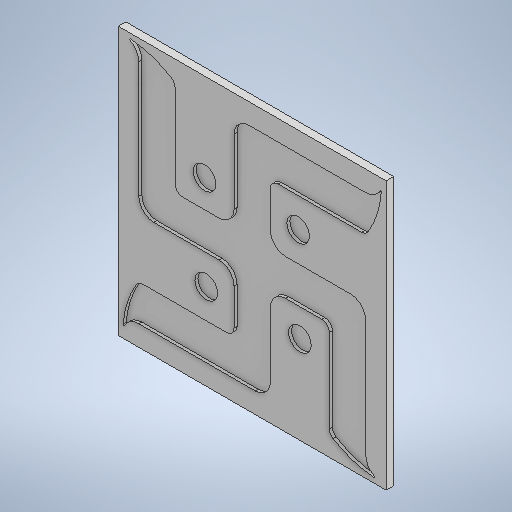
# Autodesk Inventor part: swastik@2
Saved by Autodesk Inventor 2025.2 (Build 292293000, 293)
## iProperties
Created: 2025-04-25
Part Number: swastik@2
Material: Generic
Document SubType Name: Modeling
Designer: spars
Density: 1 g/cm^3
Appearance: Default
Author: spars
Autodesk Inventor part; units mm, degrees
ref_plane "YZ Plane" through (0, 0, 0) normal (1, 0, 0) x (0, 1, 0)
ref_plane "XZ Plane" through (0, 0, 0) normal (0, 1, 0) x (-1, 0, 0)
ref_plane "XY Plane" through (0, 0, 0) normal (0, 0, 1) x (1, 0, 0)
sketch "Sketch1" plane through (0, 0, 0) normal (0, 0, 1) x (1, 0, 0)
  line L0 (75, 2) -> (75, -22)
  line L1 (-75, -2) -> (-75, 12)
  line L2 (-41, -12) -> (-65, -12)
  line L3 (-75, -2) -> (-75, 75)
  line L4 (-12, -75) -> (2, -75)
  line L5 (12, 75) -> (-2, 75)
  line L6 (75, 75) -> (-2, 75)
  line L7 (-12, 65) -> (-12, 53.1826)
  line L8 (2, -75) -> (-75, -75)
  line L9 (12, -51) -> (12, -65)
  line L10 (65, 12) -> (51, 12)
  line L11 (75, -75) -> (75, 2)
  line L12 (-75, -2) -> (-75, 75)
  line L13 (2, -75) -> (-75, -75)
  line L14 (75, 2) -> (75, -75)
  line L15 (-2, 75) -> (75, 75)
  line L16 (-51, 72.2688) -> (-51, 17)
  line L17 (51, -17) -> (51, -72.2688)
  line L18 (-72.2688, -51) -> (-17, -51)
  line L19 (17, 51) -> (72.2688, 51)
  line L20 (46, -12) -> (22, -12)
  line L21 (-22, -12) -> (-65, -12)
  line L22 (-46, 12) -> (-22, 12)
  line L23 (22, 12) -> (65, 12)
  line L24 (-12, 65) -> (-12, 22)
  line L25 (-12, -22) -> (-12, -46)
  line L26 (12, 22) -> (12, 46)
  line L27 (12, -65) -> (12, -22)
  arc A0 (-12, -22) -> (-22, -12) centre (-22, -22) ccw
  arc A1 (22, -12) -> (12, -22) centre (22, -22) ccw
  arc A2 (-22, 12) -> (-12, 22) centre (-22, 22) ccw
  arc A3 (12, 22) -> (22, 12) centre (22, 22) ccw
  arc A4 (17, 51) -> (12, 46) centre (17, 46) ccw
  arc A5 (51, -17) -> (46, -12) centre (46, -17) ccw
  arc A6 (-17, -51) -> (-12, -46) centre (-17, -46) ccw
  arc A7 (-51, 17) -> (-46, 12) centre (-46, 17) ccw
  arc A8 (75, 2) -> (65, 12) centre (65, 2) ccw
  arc A9 (-75, -2) -> (-65, -12) centre (-65, -2) ccw
  arc A10 (2, -75) -> (12, -65) centre (2, -65) ccw
  arc A11 (-2, 75) -> (-12, 65) centre (-2, 65) ccw
  circle A12 centre (-31.5, 30.3667) radius 7.5
  circle A13 centre (-30.3667, -31.5) radius 7.5
  circle A14 centre (31.5, -30.3667) radius 7.5
  circle A15 centre (30.3667, 31.5) radius 7.5
  arc A16 (-75, 75) -> (-80.7433, 84.3476) centre (-85.4787, 75) ccw
  arc A17 (-53.3988, 76.5389) -> (-80.4783, 85.2921) centre (-85.2605, 24.2339) ccw
  arc A18 (-80.4783, 85.2921) -> (-80.7433, 84.3476) centre (-80.5173, 84.7937) ccw
  arc A19 (-51, 72.2688) -> (-53.3988, 76.5389) centre (-56, 72.2688) ccw
  arc A20 (-75, -75) -> (-84.3476, -80.7433) centre (-75, -85.4787) ccw
  arc A21 (-85.2921, -80.4783) -> (-84.3476, -80.7433) centre (-84.7937, -80.5173) ccw
  arc A22 (-76.5389, -53.3988) -> (-85.2921, -80.4783) centre (-24.2339, -85.2605) ccw
  arc A23 (-72.2688, -51) -> (-76.5389, -53.3988) centre (-72.2688, -56) ccw
  arc A24 (75, -75) -> (80.7433, -84.3476) centre (85.4787, -75) ccw
  arc A25 (80.4783, -85.2921) -> (80.7433, -84.3476) centre (80.5173, -84.7937) ccw
  arc A26 (53.3988, -76.5389) -> (80.4783, -85.2921) centre (85.2605, -24.2339) ccw
  arc A27 (51, -72.2688) -> (53.3988, -76.5389) centre (56, -72.2688) ccw
  arc A28 (75, 75) -> (84.3476, 80.7433) centre (75, 85.4787) ccw
  arc A29 (85.2921, 80.4783) -> (84.3476, 80.7433) centre (84.7937, 80.5173) ccw
  arc A30 (76.5389, 53.3988) -> (85.2921, 80.4783) centre (24.2339, 85.2605) ccw
  arc A31 (72.2688, 51) -> (76.5389, 53.3988) centre (72.2688, 56) ccw
  line L28 (-72.2688, -51) -> (-72.2688, -50.8175)
  line L29 (-72.2688, -50.8175) -> (-72.1457, -50.8973)
  line L30 (-72.1457, -50.8973) -> (-72.2688, -51)
  line L31 (-88.5, 88.5) -> (88.5, 88.5)
  line L32 (88.5, 88.5) -> (88.5, -88.5)
  line L33 (88.5, -88.5) -> (-88.5, -88.5)
  line L34 (-88.5, -88.5) -> (-88.5, 88.5)
  line L35 (-88.5, 88.5) -> (88.5, -88.5) construction
  line L36 (88.5, 88.5) -> (-88.5, -88.5) construction
  point P0 (0, 0)
  dimension "d16" = 150
  dimension "d17" = 150
  dimension "d18" = 24
  dimension "d19" = 24
  dimension "d25" = 24
  dimension "d28" = 10
  dimension "d29" = 5
  dimension "d30" = 10
  dimension "d31" = 15
  dimension "d34" = 360
  dimension "d36" = 0.5
  dimension "d37" = 5
  dimension "d40" = 360
  dimension "d42" = 177
  dimension "d43" = 177
  constraints: 74 end point, 56 point on circle, 32 centre point, 30 tangent, 18 parallel, 9 equal radius, 9 perpendicular, 8 horizontal, 4 point on line, 2 midpoint, 62 other
  measures "d16" distance of L14.end L13.end
  measures "d17" distance of L6.start L14.end
  measures "d18" distance of L0.start L0.end
  measures "d19" distance of L2.end L2.start
  measures "d25" distance of L5.end L7.end
  measures "d28" radius of A0
  measures "d29" radius of A4
  measures "d30" radius of A8
  measures "d31" diameter of A12
  measures "d36" radius of A18
  measures "d37" radius of A19
  measures "d42" distance of L32.end L33.end
  measures "d43" distance of L31.end L32.end
extrude "Extrusion1" add sketch "Sketch1" along normal blind 5
extrude "Extrusion2" add sketch "Sketch1" along normal blind 3 contours L0 L11 A24 A25 A26 A27 L17 A5 L20 A1 L27 L9 A10 L4 L8 A20 A21 A22 A23 L18 A6 L25 A0 L21 L2 A9 L1 L3 A16 A18 A17 A19 L16 A7 L22 A2 L24 L7 A11 L5 L6 A28 A29 A30 A31 L19 A4 L26 A3 L23 L10 A8 | A12 | A13 | A14 | A15
body "Solid1"
